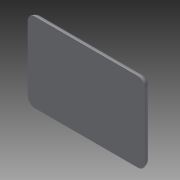
# Autodesk Inventor part: ładowarka usb v2 przykrywka
Saved by Autodesk Inventor 2014 (Build 180170000, 170)
## iProperties
Created: 2017-04-11
Part Number: ładowarka usb v2 przykrywka
Material: Ogólny
Document SubType Name: Modeling
Designer: hpdc7700
Density: 1 g/cm^3
Appearance: Domyślna
Author: hpdc7700
Autodesk Inventor part; units mm, degrees
ref_plane "YZ Plane" through (0, 0, 0) normal (1, 0, 0) x (0, 1, 0)
ref_plane "XZ Plane" through (0, 0, 0) normal (0, 1, 0) x (-1, 0, 0)
ref_plane "XY Plane" through (0, 0, 0) normal (0, 0, 1) x (1, 0, 0)
sketch "Szkic1" plane through (0, 0, 0) normal (0, 1, 0) x (-1, 0, 0)
  spline S0 degree 3 poles (16.25, 1.3463) (16.25, 1.2202) (16.2481, 1.0689) (16.2413, 0.6482) (16.2343, 0.2947) (16.2343, 0) (16.2343, -0.2947) (16.2413, -0.6482) (16.2481, -1.0689) (16.25, -1.2202) (16.25, -1.3463) knots 1.975425 1.975425 1.975425 1.975425 2.013257 2.013257 2.101653 2.101653 2.101653 2.190049 2.190049 2.22788 2.22788 2.22788 2.22788
  line L0 (16.25, 1.3463) -> (16.25, 9)
  arc A0 (16.25, 9) -> (14.25, 11) centre (14.25, 9) ccw
  line L1 (14.25, 11) -> (-14.25, 11)
  arc A1 (-14.25, 11) -> (-16.25, 9) centre (-14.25, 9) ccw
  line L2 (-16.25, 9) -> (-16.25, -9)
  arc A2 (-16.25, -9) -> (-14.25, -11) centre (-14.25, -9) ccw
  line L3 (-14.25, -11) -> (14.25, -11)
  arc A3 (14.25, -11) -> (16.25, -9) centre (14.25, -9) ccw
  line L4 (16.25, -9) -> (16.25, -1.3463)
  line L5 (-14.2536, -9) -> (-14.2536, 9)
  line L6 (-14.2536, 9) -> (14.2464, 9)
  line L7 (14.2464, 9) -> (14.2464, -9)
  line L8 (14.2464, -9) -> (-14.2536, -9)
  spline S1 degree 3 poles (16.25, 1.3463) (16.25, 1.2202) (16.2481, 1.0689) (16.2413, 0.6482) (16.2343, 0.2947) (16.2343, 0) (16.2343, -0.2947) (16.2413, -0.6482) (16.2481, -1.0689) (16.25, -1.2202) (16.25, -1.3463) knots 1.975425 1.975425 1.975425 1.975425 2.013257 2.013257 2.101653 2.101653 2.101653 2.190049 2.190049 2.22788 2.22788 2.22788 2.22788
  line L9 (16.25, 1.3463) -> (16.25, 9)
  arc A4 (16.25, 9) -> (14.25, 11) centre (14.25, 9) ccw
  line L10 (14.25, 11) -> (-14.25, 11)
  arc A5 (-14.25, 11) -> (-16.25, 9) centre (-14.25, 9) ccw
  line L11 (-16.25, 9) -> (-16.25, -9)
  arc A6 (-16.25, -9) -> (-14.25, -11) centre (-14.25, -9) ccw
  line L12 (-14.25, -11) -> (14.25, -11)
  arc A7 (14.25, -11) -> (16.25, -9) centre (14.25, -9) ccw
  line L13 (16.25, -9) -> (16.25, -1.3463)
  line L14 (-14.2536, -9) -> (-14.2536, 9)
  line L15 (-14.2536, 9) -> (14.2464, 9)
  line L16 (14.2464, 9) -> (14.2464, -9)
  line L17 (14.2464, -9) -> (-14.2536, -9)
  point P0 (0, 0)
  point P1 (0, 0)
  constraints: 36 end point, 16 point on circle, 8 centre point, 4 other
extrude "Wyciągnięcie proste1" add sketch "Szkic1" along normal blind 2 contours S0 L4 A3 L3 A2 L2 A1 L1 A0 L0 | L5 L6 L7 L8
fillet "Zaokrąglenie1" radius 2 10 edges at (15.6642, 2, 10.4142) (16.25, 2, 0) (15.6642, 2, -10.4142) (0, 2, -11) (-15.6642, 2, -10.4142) (-16.25, 2, -5.1731) (-16.2343, 2, 0) (-16.25, 2, 5.1731) (-15.6642, 2, 10.4142) (0, 2, 11)
